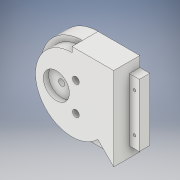
# Autodesk Inventor part: AA006b
Saved by Autodesk Inventor 2017 SP1 (Build 210196100, 196)
## iProperties
Created: 2017-06-04
Part Number: AA006b
Material: ABS Plastic
Document SubType Name: Modeling
Designer: Zach
Density: 1.06 g/cm^3
Appearance: CR White
Author: Zach
Autodesk Inventor part; units mm, degrees
ref_plane "YZ Plane" through (0, 0, 0) normal (1, 0, 0) x (0, 1, 0)
ref_plane "XZ Plane" through (0, 0, 0) normal (0, 1, 0) x (-1, 0, 0)
ref_plane "XY Plane" through (0, 0, 0) normal (0, 0, 1) x (1, 0, 0)
sketch "Sketch1" plane through (0, 0, 0) normal (0, 0, 1) x (1, 0, 0)
  line L0 (0, 0) -> (160, 0)
  line L1 (160, 0) -> (160, 160)
  line L2 (160, 160) -> (0, 160)
  line L3 (0, 160) -> (0, 0)
  circle A0 centre (50, 80) radius 6
  point P0 (160, 80)
  dimension "d0" = 160
  dimension "d1" = 160
  dimension "d2" = 12
  dimension "d7" = 50
  constraints: 8 end point, 2 parallel, 1 centre point, 1 horizontal, 1 horizontal alignment, 1 midpoint, 1 perpendicular
  measures "d0" distance of L2.end L1.end
  measures "d1" distance of L1.end L0.end
  measures "d2" diameter of A0
  measures "d7" distance from line of L3 A0.centre
extrude "Extrusion1" add sketch "Sketch1" along normal blind 50
sketch "Sketch5" plane through (0, 0, 50) normal (0, 0, 1) x (1, 0, 0)
  circle A0 centre (50, 80) radius 6 projected
  line L0 (0, 0) -> (160, 0) projected
  line L1 (160, 0) -> (160, 160) projected
  line L2 (160, 160) -> (0, 160) projected
  line L3 (0, 160) -> (0, 0) projected
  circle A1 centre (80, 80) radius 80 construction
  line L4 (0, 0) -> (160, 0) projected
  arc A2 (80, 160) -> (80, 0) centre (80, 80) ccw
  line L5 (160, 160) -> (0, 160) projected
  line L6 (80, 160) -> (0, 160)
  line L7 (0, 160) -> (0, 0)
  line L8 (80, 0) -> (0, 0)
  point P0 (0, 80)
  constraints: 6 end point, 4 point on circle, 4 tangent, 3 midpoint, 2 centre point, 2 collinear, 1 horizontal alignment, 1 perpendicular
extrude "Extrusion5" cut sketch "Sketch5" against normal through all contours L3 A2 L0 | L3 L2 A2
sketch "Sketch17" plane through (0, 0, 50) normal (0, 0, 1) x (1, 0, 0)
  circle A0 centre (50, 80) radius 6 projected
  circle A1 centre (50, 80) radius 6 projected
  circle A2 centre (50, 80) radius 25
  point P0 (0, 0)
  dimension "d80" = 50
  constraints: 1 centre point, 1 coincident
  measures "d80" diameter of A2
extrude "Extrusion17" cut sketch "Sketch17" against normal blind 10
sketch "Sketch18" plane through (0, 0, 0) normal (0, 0, -1) x (-1, 0, 0)
  circle A0 centre (-50, 80) radius 6 projected
  point P0 (0, 0)
extrude "Extrusion18" add sketch "Sketch18" against normal blind 12.5
sketch "Sketch19" plane through (0, 0, 0) normal (0, 0, -1) x (-1, 0, 0)
  line L0 (-160, 0) -> (-160, 160) projected
  line L1 (-160, 20) -> (-179, 20)
  line L2 (-179, 20) -> (-179, 140)
  line L3 (-179, 140) -> (-160, 140)
  line L4 (-160, 140) -> (-160, 20)
  line L5 (-80, 0) -> (-160, 0) projected
  line L6 (-160, 160) -> (-80, 160) projected
  circle A0 centre (-170, 42.5) radius 2.5
  line L7 (-170, 42.5) -> (-170, 117.5) construction
  circle A1 centre (-170, 117.5) radius 2.5
  point P0 (0, 0)
  point P1 (-160, 80)
  point P2 (-170, 80)
  point P3 (-160, 80)
  dimension "d85" = 19
  dimension "d86" = 20
  dimension "d87" = 20
  dimension "d88" = 5
  dimension "d89" = 10
  dimension "d100" = 75
  dimension "d101" = 5
  constraints: 10 end point, 3 midpoint, 2 centre point, 2 parallel, 1 coincident, 1 horizontal, 1 horizontal alignment, 1 perpendicular, 1 point on line, 1 vertical
  measures "d85" distance of L2.end L3.end
  measures "d86" distance between parallel lines of L1 L5
  measures "d87" distance between parallel lines of L6 L3
  measures "d88" diameter of A0
  measures "d89" distance from line of L0 L7.start
  measures "d100" distance of L7.start L7.end
  measures "d101" diameter of A1
extrude "Extrusion19" add sketch "Sketch19" against normal blind 20
sketch "Sketch20" plane through (0, 0, 0) normal (0, 0, -1) x (-1, 0, 0)
  circle A0 centre (-170, 42.5) radius 2.5 projected
  circle A1 centre (-170, 42.5) radius 6.5
  circle A2 centre (-170, 117.5) radius 2.5 projected
  circle A3 centre (-170, 117.5) radius 6.5
  point P0 (0, 0)
  dimension "d92" = 13
  dimension "d102" = 13
  constraints: 2 centre point, 2 coincident
  measures "d92" diameter of A1
  measures "d102" diameter of A3
extrude "Extrusion20" cut sketch "Sketch20" against normal blind 15 contours A0 | A1 | A3
sketch "Sketch21" plane through (0, 0, 0) normal (0, 0, -1) x (-1, 0, 0)
  circle A0 centre (-170, 42.5) radius 6.5 projected
  arc A1 (-80, 0) -> (-80, 160) centre (-80, 80) ccw projected
  line L0 (-160, 160) -> (-80, 160) projected
  line L1 (-160, 140) -> (-160, 160) projected
  line L2 (-179, 140) -> (-160, 140) projected
  line L3 (-179, 20) -> (-179, 140) projected
  line L4 (-160, 20) -> (-179, 20) projected
  line L5 (-160, 0) -> (-160, 20) projected
  line L6 (-80, 0) -> (-160, 0) projected
  circle A2 centre (-50, 80) radius 6 construction
  arc A3 (-80, 10) -> (-80, 150) centre (-80, 80) ccw construction
  line L7 (-80, 10) -> (-150, 10)
  line L8 (-150, 10) -> (-150, 30)
  line L9 (-150, 30) -> (-169, 30) construction
  line L10 (-169, 30) -> (-169, 130) construction
  line L11 (-169, 130) -> (-150, 130) construction
  line L12 (-150, 130) -> (-150, 150)
  line L13 (-150, 150) -> (-80, 150)
  line L14 (-150, 130) -> (-150, 30) construction
  line L15 (-150, 72.5) -> (-73.8485, 72.5)
  line L16 (-111.9242, 72.5) -> (-111.9242, 87.5) construction
  line L17 (-150, 87.5) -> (-73.8485, 87.5)
  line L18 (-150, 130) -> (-150, 87.5)
  line L19 (-150, 30) -> (-150, 72.5)
  line L20 (-26.1515, 72.5) -> (-10.4029, 72.5)
  line L21 (-26.1515, 87.5) -> (-10.4029, 87.5)
  line L22 (-57.5, 103.8485) -> (-57.5, 146.2854)
  line L23 (-42.5, 103.8485) -> (-42.5, 139.108)
  line L24 (-57.5, 121.4782) -> (-42.5, 121.4782) construction
  line L25 (-42.5, 56.1515) -> (-42.5, 20.892)
  line L26 (-57.5, 56.1515) -> (-57.5, 13.7146)
  circle A4 centre (-50, 80) radius 25 construction
  arc A5 (-57.5, 146.2854) -> (-80, 150) centre (-80, 80) ccw
  arc A6 (-10.4029, 87.5) -> (-42.5, 139.108) centre (-80, 80) ccw
  arc A7 (-42.5, 20.892) -> (-10.4029, 72.5) centre (-80, 80) ccw
  arc A8 (-80, 10) -> (-57.5, 13.7146) centre (-80, 80) ccw
  arc A9 (-57.5, 103.8485) -> (-73.8485, 87.5) centre (-50, 80) ccw
  arc A10 (-26.1515, 87.5) -> (-42.5, 103.8485) centre (-50, 80) ccw
  arc A11 (-42.5, 56.1515) -> (-26.1515, 72.5) centre (-50, 80) ccw
  arc A12 (-73.8485, 72.5) -> (-57.5, 56.1515) centre (-50, 80) ccw
  point P0 (0, 0)
  point P1 (-111.9242, 80)
  point P2 (-50, 121.4782)
  dimension "d95" = 10
  dimension "d96" = 15
  dimension "d99" = 15
  constraints: 40 end point, 27 point on circle, 9 centre point, 9 concentric, 5 midpoint, 5 vertical, 3 horizontal, 3 horizontal alignment, 3 point on line, 3 vertical alignment, 2 collinear, 2 parallel, 1 perpendicular, 7 other
  measures "d95" distance between parallel lines of L0 L13
  measures "d96" distance of L16.end L16.start
  measures "d99" distance of L24.end L24.start
extrude "Extrusion21" cut sketch "Sketch21" against normal blind 40 contours L7 L8 L19 L15 A12 L26 A8 | L12 L13 A5 L22 A9 L17 L18 | L20 A7 L25 A11 | A10 L23 A6 L21
sketch "Sketch23" plane through (0, 0, 50) normal (0, 0, 1) x (1, 0, 0)
  circle A0 centre (87.5, 52.5) radius 2.5
  circle A1 centre (87.5, 107.5) radius 2.5
  line L0 (160, 0) -> (160, 160) construction
  line L1 (87.5, 52.5) -> (87.5, 107.5) construction
  point P0 (0, 0)
  point P1 (87.5, 80)
  point P2 (160, 80)
  dimension "d103" = 5
  dimension "d104" = 5
  dimension "d105" = 55
  dimension "d106" = 72.5
  constraints: 2 centre point, 2 end point, 2 midpoint, 1 horizontal alignment, 1 vertical, 1 vertical alignment
  measures "d103" diameter of A0
  measures "d104" diameter of A1
  measures "d105" distance of L1.start L1.end
  measures "d106" distance from line of L0 L1.start
extrude "Extrusion22" cut sketch "Sketch23" against normal through all
sketch "Sketch24" plane through (0, 0, 40) normal (0, 0, -1) x (-1, 0, 0)
  line L0 (-95, 150) -> (-95, 10)
  line L1 (-80, 150) -> (-80, 10)
  line L2 (-80, 150) -> (-95, 150)
  line L3 (-95, 10) -> (-80, 10)
  line L4 (-95, 80) -> (-80, 80) construction
  circle A0 centre (-87.5, 107.5) radius 2.5 projected
  circle A1 centre (-87.5, 52.5) radius 2.5 projected
  point P0 (0, 0)
  point P1 (-87.5, 80)
  point P2 (-87.5, 10)
  point P3 (-150, 150)
  point P4 (-150, 10)
  dimension "d110" = 15
  constraints: 10 end point, 4 horizontal alignment, 4 midpoint, 2 horizontal, 2 vertical, 1 vertical alignment
  measures "d110" distance of L4.start L4.end
extrude "Extrusion23" add sketch "Sketch24" along normal blind 40
sketch "Sketch26" plane through (0, 0, 50) normal (0, 0, 1) x (1, 0, 0)
  circle A0 centre (87.5, 107.5) radius 2.5 projected
  circle A1 centre (87.5, 52.5) radius 2.5 projected
  circle A2 centre (87.5, 52.5) radius 6.5
  circle A3 centre (87.5, 107.5) radius 6.5
  point P0 (0, 0)
  dimension "d115" = 13
  dimension "d116" = 13
  constraints: 2 centre point, 2 coincident
  measures "d115" diameter of A2
  measures "d116" diameter of A3
extrude "Extrusion24" cut sketch "Sketch26" against normal blind 30 contours A0 | A1 | A2 | A3
sketch "Sketch27" plane through (0, 0, 50) normal (0, 0, 1) x (1, 0, 0)
  arc A0 (80, 160) -> (80, 0) centre (80, 80) ccw construction
  circle A1 centre (80, 80) radius 80 construction
  circle A2 centre (80, 80) radius 70 construction
  line L0 (80, 0) -> (160, 0) projected
  line L1 (160, 160) -> (80, 160) projected
  arc A3 (80, 160) -> (80, 0) centre (80, 80) ccw projected
  arc A4 (80, 160) -> (80, 160) centre (80, 80) ccw
  line L2 (80, 160) -> (80, 150)
  arc A5 (80, 150) -> (57.5, 146.2854) centre (80, 80) ccw projected
  line L3 (160, 0) -> (129.4975, 30.5025)
  line L4 (160, 0) -> (80, 80) construction
  arc A6 (80, 150) -> (57.5, 146.2854) centre (80, 80) ccw projected
  arc A7 (80, 150) -> (129.4975, 30.5025) centre (80, 80) ccw
  point P0 (0, 0)
  point P1 (160, 80)
  point P2 (150, 80)
  dimension "d119" = 10
  constraints: 6 end point, 6 point on circle, 3 centre point, 1 coincident, 1 concentric, 1 point on line, 1 vertical, 1 vertical alignment, 3 other
  measures "d119" radial gap between concentric circles of A1 A2
extrude "Extrusion25" cut sketch "Sketch27" against normal blind 20 contours A4 L3 L0 | A3 L2 A5 A7 L3 A4
sketch "Sketch30" plane through (0, 0, 30) normal (0, 0, 1) x (1, 0, 0)
  line L0 (95, 10) -> (150, 10) projected
  line L1 (95, 11.626) -> (95, 10) projected
  line L2 (129.4975, 30.5025) -> (160, 0) construction
  arc A0 (80, 150) -> (129.4975, 30.5025) centre (80, 80) ccw construction
  arc A1 (95, 11.626) -> (129.4975, 30.5025) centre (80, 80) ccw
  line L3 (150, 10) -> (129.4975, 30.5025)
  point P0 (0, 0)
  constraints: 2 end point, 2 point on circle, 1 centre point, 1 concentric
extrude "Extrusion28" add sketch "Sketch30" against normal blind 5
sketch "Sketch31" plane through (0, 0, 40) normal (0, 0, -1) x (-1, 0, 0)
  arc A0 (-129.4975, 30.5025) -> (-95, 11.626) centre (-80, 80) ccw projected
  line L0 (-129.4975, 30.5025) -> (-150, 10) projected
  arc A1 (-80, 10) -> (-57.5, 13.7146) centre (-80, 80) ccw projected
  arc A2 (-129.4975, 30.5025) -> (-80, 150) centre (-80, 80) ccw projected
  arc A3 (-129.3613, 37.7098) -> (-80, 145) centre (-80, 80) ccw
  line L1 (-80, 150) -> (-80, 145)
  line L2 (-129.3613, 37.7098) -> (-153.5355, 13.5355)
  line L3 (-129.3613, 37.7098) -> (-129.3363, 37.7348)
  line L4 (-150, 10) -> (-153.5355, 13.5355)
  point P0 (0, 0)
  dimension "d130" = 5
  dimension "d131" = 5
  constraints: 8 end point, 2 point on circle, 1 centre point, 1 parallel, 1 perpendicular, 1 vertical
  measures "d130" radial gap between concentric circles of A2 A3
  measures "d131" distance between parallel lines of L0 L2
extrude "Extrusion29" add sketch "Sketch31" along normal blind 15
body "Solid1"
